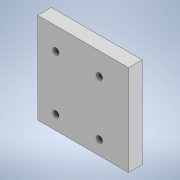
# Autodesk Inventor part: 20220509_知能ロボットキャスタ
Saved by Autodesk Inventor 2020 (Build 240168000, 168)
## iProperties
Created: 2022-05-08
Part Number: 20220509_知能ロボットキャスタ
Material: 一般
Document SubType Name: Modeling
Designer: Naggy
Density: 1 g/cm^3
Appearance: 既定
Author: Naggy
Autodesk Inventor part; units mm, degrees
ref_plane "YZ Plane" through (0, 0, 0) normal (1, 0, 0) x (0, 1, 0)
ref_plane "XZ Plane" through (0, 0, 0) normal (0, 1, 0) x (-1, 0, 0)
ref_plane "XY Plane" through (0, 0, 0) normal (0, 0, 1) x (1, 0, 0)
sketch "スケッチ1" plane through (0, 0, 0) normal (0, 0, 1) x (1, 0, 0)
  line L0 (-25, -25) -> (25, -25)
  line L1 (25, -25) -> (25, 25)
  line L2 (25, 25) -> (-25, 25)
  line L3 (-25, 25) -> (-25, -25)
  line L4 (-25, -25) -> (25, 25) construction
  line L5 (25, -25) -> (-25, 25) construction
  point P0 (0, 0)
  dimension "d0" = 50
  dimension "d1" = 50
  constraints: 12 end point, 2 midpoint, 2 parallel, 1 horizontal, 1 perpendicular
  measures "d0" distance between parallel lines of L0 L2
  measures "d1" distance between parallel lines of L1 L3
extrude "押し出し1" add sketch "スケッチ1" along normal blind 7.5
sketch "スケッチ2" plane through (0, 0, 7.5) normal (0, 0, 1) x (1, 0, 0)
  line L0 (-25, 25) -> (-25, -25) projected
  line L1 (-25, -25) -> (25, -25) projected
  point P0 (0, 0)
  point P1 (-15, 12.836)
  point P2 (9, 12.836)
  point P3 (9, -17.164)
  point P4 (-15, -17.164)
  dimension "d4" = 10
  dimension "d5" = 10
  dimension "d6" = 30
  dimension "d7" = 30
  dimension "d8" = 24
  dimension "d16" = 7.836
  dimension "d17" = 7.836
  measures "d4" distance from line of point (-15, 12.836) L0
  measures "d5" distance from line of point (-15, -17.164) L0
  measures "d6" distance of point (-15, -17.164) point (-15, 12.836)
  measures "d7" distance of point (9, 12.836) point (9, -17.164)
  measures "d8" distance of point (9, 12.836) point (-15, 12.836)
  measures "d16" distance from line of L1 point (-15, -17.164)
  measures "d17" distance from line of L1 point (9, -17.164)
hole "穴1" at (-15, 12.836, 7.5) at (9, 12.836, 7.5) at (9, -17.164, 7.5) at (-15, -17.164, 7.5) direction (0, 0, -1) diameter 3.4 end through all clearance for "Flat Head Machine Screw" size "M3" standard "Ansi Metric M Profile"
